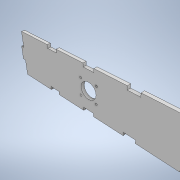
# Autodesk Inventor part: Стекнка t2
Saved by Autodesk Inventor 2021 (Build 250183000, 183)
## iProperties
Created: 2021-04-10
Part Number: Стекнка t2
Material: Типовые
Document SubType Name: Modeling
Designer: user
Density: 1 g/cm^3
Appearance: По умолчанию
Author: user
Autodesk Inventor part; units mm, degrees
ref_plane "YZ Plane" through (0, 0, 0) normal (1, 0, 0) x (0, 1, 0)
ref_plane "XZ Plane" through (0, 0, 0) normal (0, 1, 0) x (-1, 0, 0)
ref_plane "XY Plane" through (0, 0, 0) normal (0, 0, 1) x (1, 0, 0)
sketch "Эскиз1" plane through (0, 0, 0) normal (0, 0, 1) x (1, 0, 0)
  line L0 (-74.9994, 20) -> (-42.5, 20)
  line L1 (-32.5, 20) -> (-32.5, 17)
  line L2 (-32.5, 17) -> (-42.5, 17)
  line L3 (-42.5, 17) -> (-42.5, 20)
  line L4 (-32.5, 20) -> (-5, 20)
  line L5 (0, 17) -> (-5, 17)
  line L6 (-5, 17) -> (-5, 20)
  line L7 (-74.9994, 6.0502) -> (-77.9994, 6.0502)
  line L8 (-74.9994, 20) -> (-42.5, 20)
  line L9 (-32.5, 20) -> (-5, 20)
  line L10 (75.0067, 20) -> (42.5, 20)
  line L11 (32.5, 20) -> (32.5, 17)
  line L12 (32.5, 17) -> (42.5, 17)
  line L13 (42.5, 17) -> (42.5, 20)
  line L14 (32.5, 20) -> (5, 20)
  line L15 (0, 17) -> (5, 17)
  line L16 (5, 17) -> (5, 20)
  line L17 (75.0067, 5.8458) -> (78.0067, 5.8458)
  line L18 (75.0067, 20) -> (42.5, 20)
  line L19 (32.5, 20) -> (5, 20)
  line L20 (-74.9994, -20) -> (-42.5, -20)
  line L21 (-32.5, -20) -> (-32.5, -17)
  line L22 (-32.5, -17) -> (-42.5, -17)
  line L23 (-42.5, -17) -> (-42.5, -20)
  line L24 (-32.5, -20) -> (-5, -20)
  line L25 (-32.5, -20) -> (-5, -20)
  line L26 (-74.9994, -5.9498) -> (-77.9994, -5.9498)
  line L27 (-74.9994, -20) -> (-42.5, -20)
  line L28 (-5, -17) -> (-5, -20)
  line L29 (0, -17) -> (-5, -17)
  line L30 (0, -17) -> (5, -17)
  line L31 (32.5, -20) -> (32.5, -17)
  line L32 (32.5, -20) -> (5, -20)
  line L33 (32.5, -20) -> (5, -20)
  line L34 (32.5, -17) -> (42.5, -17)
  line L35 (42.5, -17) -> (42.5, -20)
  line L36 (75.0067, -20) -> (42.5, -20)
  line L37 (75.0067, -20) -> (42.5, -20)
  line L38 (75.0067, -6.1542) -> (78.0067, -6.1542)
  line L39 (5, -17) -> (5, -20)
  line L40 (-74.9994, 6.0502) -> (-74.9994, 20)
  line L41 (-74.9994, -5.9498) -> (-74.9994, -20)
  line L42 (-74.9994, 6.0502) -> (-77.9994, 6.0502)
  line L43 (-77.9994, 6.0502) -> (-77.9994, -5.9498)
  line L44 (-77.9994, -5.9498) -> (-74.9994, -5.9498)
  line L45 (75.0067, 20) -> (75.0067, 5.8458)
  line L46 (75.0067, -6.1542) -> (75.0067, -20)
  line L47 (75.0067, 5.8458) -> (78.0067, 5.8458)
  line L48 (78.0067, 5.8458) -> (78.0067, -6.1542)
  line L49 (78.0067, -6.1542) -> (75.0067, -6.1542)
  circle A0 centre (0, 0) radius 7.25
  circle A1 centre (-7.5, -7.5) radius 1
  circle A2 centre (7.5, -7.5) radius 1
  circle A3 centre (7.5, 7.5) radius 1
  circle A4 centre (-7.5, 7.5) radius 1
  constraints: 100 end point, 5 centre point, 4 horizontal, 3 parallel, 3 perpendicular, 2 point on line, 1 coincident
extrude "Выдавливание1" add sketch "Эскиз1" along normal blind 3
